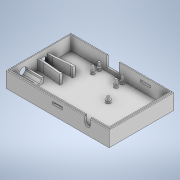
# Autodesk Inventor part: Housing
Saved by Autodesk Inventor 2020 (Build 240168000, 168)
## iProperties
Created: 2019-10-15
Part Number: Housing
Material: Generic
Document SubType Name: Modeling
Designer: strom
Density: 1 g/cm^3
Appearance: Default
Author: strom
Autodesk Inventor part; units mm, degrees
ref_plane "YZ Plane" through (0, 0, 0) normal (1, 0, 0) x (0, 1, 0)
ref_plane "XZ Plane" through (0, 0, 0) normal (0, 1, 0) x (-1, 0, 0)
ref_plane "XY Plane" through (0, 0, 0) normal (0, 0, 1) x (1, 0, 0)
sketch "Sketch1" plane through (0, 0, 0) normal (0, 1, 0) x (-1, 0, 0)
  line L0 (68.58, -43.18) -> (-68.58, -43.18)
  line L1 (-68.58, -43.18) -> (-68.58, 43.18)
  line L2 (-68.58, 43.18) -> (68.58, 43.18)
  line L3 (68.58, 43.18) -> (68.58, -43.18)
  line L4 (96.012, 0) -> (-96.012, 0) projected
  line L5 (0, -60.452) -> (0, 60.452) projected
  point P0 (0, 0)
  dimension "d0" = 137.16
  dimension "d1" = 86.36
  constraints: 8 end point, 2 parallel, 1 horizontal, 1 perpendicular, 2 other
  measures "d0" distance of L1.end L2.end
  measures "d1" distance of L0.end L1.end
extrude "Extrusion1" add sketch "Sketch1" along normal blind 21.59
shell "Shell1" thickness 2.54 removed faces 1 at (-22.86, 21.59, -14.3933)
sketch "Sketch2" plane through (-66.04, 2.54, 40.64) normal (0, 1, 0) x (1, 0, 0)
  line L0 (-29.972, 40.64) -> (162.052, 40.64) projected
  line L1 (66.04, 101.092) -> (66.04, -19.812) projected
  circle A0 centre (83.82, 47.2821) radius 3.175
  circle A1 centre (127, 47.2821) radius 3.175
  circle A2 centre (83.82, 4.1021) radius 3.175
  circle A3 centre (127, 4.1021) radius 3.175
  line L2 (132.08, 0) -> (0, 0) projected
  line L3 (132.08, 81.28) -> (132.08, 0) projected
  point P0 (66.04, 40.64)
  dimension "d5" = 6.35
  dimension "d6" = 6.35
  dimension "d7" = 6.35
  dimension "d8" = 6.35
  dimension "d9" = 43.18
  dimension "d10" = 43.18
  dimension "d11" = 4.1021
  dimension "d22" = 5.08
  constraints: 4 centre point, 2 horizontal alignment, 2 vertical alignment
  measures "d5" diameter of A0
  measures "d6" diameter of A1
  measures "d7" diameter of A3
  measures "d8" diameter of A2
  measures "d9" distance of A1.centre A0.centre
  measures "d10" distance of A2.centre A0.centre
  measures "d11" distance from line of L2 A2.centre
  measures "d22" distance from line of L3 A1.centre
extrude "Extrusion2" add sketch "Sketch2" along normal blind 3.048 contours A0 | A1 | A2 | A3
sketch "Sketch3" plane through (17.78, 5.588, -6.6421) normal (0, 1, 0) x (1, 0, 0)
  circle A0 centre (0, 0) radius 3.175 projected
  circle A1 centre (43.18, 0) radius 3.175 projected
  circle A2 centre (43.18, -43.18) radius 3.175 projected
  circle A3 centre (0, -43.18) radius 3.175 projected
  circle A4 centre (0, 0) radius 3.175 projected
  circle A5 centre (0, 0) radius 1.524
  circle A6 centre (43.18, 0) radius 1.524
  circle A7 centre (0, -43.18) radius 3.175 projected
  circle A8 centre (0, -43.18) radius 1.524
  circle A9 centre (43.18, -43.18) radius 1.524
  point P0 (-17.78, -6.6421)
  dimension "d14" = 3.048
  dimension "d15" = 3.048
  dimension "d16" = 3.048
  dimension "d17" = 3.048
  constraints: 4 centre point, 4 coincident
  measures "d14" diameter of A5
  measures "d15" diameter of A6
  measures "d16" diameter of A9
  measures "d17" diameter of A8
extrude "Extrusion3" add sketch "Sketch3" along normal blind 3.81 contours A5 | A6 | A8 | A9
sketch "Sketch4" plane through (-68.58, 0, 43.18) normal (0, 0, 1) x (1, 0, 0)
  line L0 (89.535, 5.588) -> (83.185, 5.588) projected
  line L1 (83.185, 2.54) -> (89.535, 2.54) projected
  line L2 (132.715, 5.588) -> (126.365, 5.588) projected
  line L3 (126.365, 2.54) -> (132.715, 2.54) projected
  circle A0 centre (108.6485, 13.208) radius 3.6195
  line L4 (87.884, 9.398) -> (84.836, 9.398) projected
  line L5 (84.836, 5.588) -> (87.884, 5.588) projected
  line L6 (128.016, 5.588) -> (131.064, 5.588) projected
  line L7 (131.064, 9.398) -> (128.016, 9.398) projected
  line L8 (128.016, 5.588) -> (131.064, 5.588) projected
  line L9 (105.029, 13.208) -> (105.029, 21.59)
  line L10 (112.268, 13.208) -> (112.268, 21.59)
  line L11 (0, 21.59) -> (137.16, 21.59) projected
  point P0 (68.58, 0)
  dimension "d20" = 7.239
  dimension "d23" = 20.7645
  dimension "d24" = 7.62
  constraints: 4 end point, 2 point on circle, 2 point on line, 2 tangent, 2 vertical, 1 centre point
  measures "d20" diameter of A0
  measures "d23" horizontal distance of A0.centre L4.start
  measures "d24" distance from line of A0.centre L0
extrude "Extrusion4" cut sketch "Sketch4" against normal blind 3.81
sketch "Sketch5" plane through (-66.04, 2.54, 40.64) normal (0, 1, 0) x (1, 0, 0)
  circle A0 centre (127, 4.1021) radius 3.175 projected
  circle A1 centre (127, 47.2821) radius 3.175 projected
  circle A2 centre (83.82, 4.1021) radius 3.175 projected
  circle A3 centre (83.82, 47.2821) radius 3.175 projected
  line L0 (0, 0) -> (132.08, 0) projected
  line L1 (132.08, 0) -> (132.08, 81.28) projected
  line L2 (132.08, 81.28) -> (0, 81.28) projected
  line L3 (0, 81.28) -> (0, 0) projected
  line L4 (0, 25.4) -> (19.05, 25.4)
  line L5 (19.05, 25.4) -> (19.05, 10.16)
  line L6 (19.05, 10.16) -> (0, 10.16)
  line L7 (0, 10.16) -> (0, 25.4)
  line L8 (0, 0) -> (0, 81.28) projected
  point P0 (66.04, 40.64)
  point P1 (0, 25.4)
  point P2 (0, 10.16)
  dimension "d27" = 19.05
  dimension "d28" = 15.24
  dimension "d29" = 10.16
  constraints: 8 end point, 2 parallel, 1 collinear, 1 horizontal, 1 perpendicular
  measures "d27" distance of L5.end L6.end
  measures "d28" distance of L4.end L5.end
  measures "d29" distance between parallel lines of L6 L0
extrude "Extrusion5" add sketch "Sketch5" along normal blind 7.62 contours L3 L4 L5 L6
sketch "Sketch6" plane through (-46.99, 2.54, 30.48) normal (1, 0, 0) x (0, 0, -1)
  line L0 (0, 7.62) -> (15.24, 7.62) projected
  line L1 (5.4106, 2.286) -> (2.286, 5.4106)
  line L2 (2.286, 5.4106) -> (2.286, 9.8294)
  line L3 (2.286, 9.8294) -> (5.4106, 12.954)
  line L4 (5.4106, 12.954) -> (9.8294, 12.954)
  line L5 (9.8294, 12.954) -> (12.954, 9.8294)
  line L6 (12.954, 9.8294) -> (12.954, 5.4106)
  line L7 (12.954, 5.4106) -> (9.8294, 2.286)
  line L8 (9.8294, 2.286) -> (5.4106, 2.286)
  point P0 (30.48, -2.54)
  point P1 (7.62, 7.62)
  dimension "d34" = 10.668
  constraints: 16 end point, 1 horizontal, 1 midpoint, 17 other
  measures "d34" distance between parallel lines of L6 L2
extrude "Extrusion6" cut sketch "Sketch6" against normal through all
sketch "Sketch7" plane through (-46.99, 2.54, 15.24) normal (0, 0, -1) x (-1, 0, 0)
  line L0 (0, 0) -> (19.05, 0) projected
  line L1 (0, 0) -> (0, 7.62) projected
  line L2 (19.05, 7.62) -> (0, 7.62) projected
  line L3 (19.05, 0) -> (19.05, 7.62) projected
  line L4 (0, 0) -> (19.05, 0) projected
  line L5 (2.54, 0) -> (6.35, 0)
  line L6 (6.35, 0) -> (6.35, 1.905)
  line L7 (6.35, 1.905) -> (2.54, 1.905)
  line L8 (2.54, 1.905) -> (2.54, 0)
  line L9 (12.7, 0) -> (16.51, 0)
  line L10 (16.51, 0) -> (16.51, 1.905)
  line L11 (16.51, 1.905) -> (12.7, 1.905)
  line L12 (12.7, 1.905) -> (12.7, 0)
  point P0 (-46.99, -2.54)
  point P1 (16.51, 0)
  point P2 (2.54, 0)
  point P3 (6.35, 0)
  dimension "d37" = 3.81
  dimension "d38" = 1.905
  dimension "d39" = 3.81
  dimension "d40" = 1.905
  dimension "d41" = 2.54
  dimension "d42" = 2.54
  constraints: 16 end point, 4 parallel, 2 horizontal, 2 perpendicular, 2 point on line
  measures "d37" distance of L7.end L6.end
  measures "d38" distance between parallel lines of L0 L7
  measures "d39" distance of L11.end L10.end
  measures "d40" distance of L10.end L9.end
  measures "d41" distance between parallel lines of L10 L3
  measures "d42" distance between parallel lines of L1 L8
extrude "Extrusion7" cut sketch "Sketch7" against normal up to surface (15.24 mm away) contours L8 L7 L6 L0 | L12 L11 L10 L0
sketch "Sketch8" plane through (-66.04, 2.54, 40.64) normal (0, 1, 0) x (1, 0, 0)
  line L0 (0, 81.28) -> (0, 25.4) projected
  line L1 (0, 39.37) -> (7.62, 39.37)
  line L2 (7.62, 39.37) -> (29.718, 37.2111)
  line L3 (29.718, 37.2111) -> (29.718, 37.7191)
  line L4 (29.718, 37.7191) -> (32.258, 37.7191)
  line L5 (32.258, 37.7191) -> (32.258, 34.4108)
  line L6 (32.258, 34.4108) -> (7.4962, 36.83)
  line L7 (7.4962, 36.83) -> (0, 36.83)
  line L8 (0, 49.53) -> (7.62, 49.53)
  line L9 (7.62, 49.53) -> (29.718, 51.6891)
  line L10 (29.718, 51.6891) -> (29.718, 51.1811)
  line L11 (29.718, 51.1811) -> (32.258, 51.1811)
  line L12 (32.258, 51.1811) -> (32.258, 54.4893)
  line L13 (0, 0) -> (0, 81.28) projected
  line L14 (32.258, 54.4893) -> (7.4962, 52.07)
  line L15 (7.4962, 52.07) -> (0, 52.07)
  line L16 (19.05, 25.4) -> (0, 25.4) projected
  point P0 (66.04, 40.64)
  point P1 (0, 54.9166)
  point P2 (0, 54.9166)
  dimension "d45" = 7.62
  dimension "d46" = 7.62
  dimension "d47" = 10.16
  dimension "d48" = 14.478
  dimension "d49" = 22.098
  dimension "d50" = 22.098
  dimension "d51" = 0.508
  dimension "d52" = 0.508
  dimension "d53" = 2.54
  dimension "d54" = 2.54
  dimension "d55" = 2.54
  dimension "d56" = 2.54
  dimension "d57" = 2.54
  dimension "d58" = 2.54
  dimension "d59" = 11.43
  dimension "d60" = 5.58
  constraints: 28 end point, 6 perpendicular, 4 horizontal, 4 point on line, 2 parallel, 1 coincident, 1 vertical, 5 other
  measures "d45" distance of L1.start L1.end
  measures "d46" distance from line of L8.end L0
  measures "d47" distance between parallel lines of L1 L8
  measures "d48" distance of L9.end L2.end
  measures "d49" distance from line of L3 L1.end
  measures "d50" distance from line of L10 L8.end
  measures "d51" distance of L2.end L3.end
  measures "d52" distance of L9.end L10.end
  measures "d53" distance between parallel lines of L1 L7
  measures "d54" distance between parallel lines of L15 L8
  measures "d55" distance between parallel lines of L2 L6
  measures "d56" distance between parallel lines of L14 L9
  measures "d57" distance between parallel lines of L3 L5
  measures "d58" distance between parallel lines of L10 L12
  measures "d59" distance between parallel lines of L16 L7
  measures "d60" angle of L1 L2
extrude "Extrusion8" add sketch "Sketch8" along normal blind 12.7
sketch "Sketch9" plane through (-66.04, 2.54, -40.64) normal (1, 0, 0) x (0, 0, -1)
  line L0 (-41.91, 12.7) -> (-41.91, 0) projected
  line L1 (-31.75, 0) -> (-31.75, 12.7) projected
  circle A0 centre (-36.83, 6.096) radius 5.08
  line L2 (2.54, -2.54) -> (-83.82, -2.54) projected
  point P0 (-40.64, -2.54)
  dimension "d63" = 10.16
  dimension "d64" = 8.636
  constraints: 1 centre point, 1 tangent
  measures "d63" diameter of A0
  measures "d64" distance from line of L2 A0.centre
extrude "Extrusion9" cut sketch "Sketch9" against normal blind 12.7
sketch "Sketch10" plane through (-66.04, 2.54, 40.64) normal (0, 1, 0) x (1, 0, 0)
  line L0 (0, 81.28) -> (132.08, 81.28) projected
  circle A0 centre (40.64, 78.232) radius 2.54
  circle A1 centre (40.64, 69.85) radius 2.54
  circle A2 centre (71.5518, 78.232) radius 2.54
  circle A3 centre (71.5518, 69.85) radius 2.54
  line L1 (0, 0) -> (0, 81.28) projected
  point P0 (66.04, 40.64)
  dimension "d67" = 5.08
  dimension "d68" = 5.08
  dimension "d69" = 5.08
  dimension "d70" = 5.08
  dimension "d71" = 30.9118
  dimension "d72" = 30.9118
  dimension "d73" = 8.382
  dimension "d74" = 8.382
  dimension "d75" = 3.048
  dimension "d76" = 40.64
  constraints: 4 centre point, 1 horizontal alignment, 1 vertical alignment
  measures "d67" diameter of A0
  measures "d68" diameter of A1
  measures "d69" diameter of A2
  measures "d70" diameter of A3
  measures "d71" distance of A2.centre A0.centre
  measures "d72" distance of A3.centre A1.centre
  measures "d73" distance of A0.centre A1.centre
  measures "d74" distance of A3.centre A2.centre
  measures "d75" distance from line of L0 A0.centre
  measures "d76" distance from line of L1 A0.centre
extrude "Extrusion10" add sketch "Sketch10" along normal blind 4.445
sketch "Sketch11" plane through (-66.04, 2.54, -40.64) normal (0, 0, 1) x (1, 0, 0)
  line L0 (43.18, 4.445) -> (38.1, 4.445) projected
  line L1 (38.1, 0) -> (43.18, 0) projected
  line L2 (43.18, 0) -> (43.18, 4.445) projected
  line L3 (38.1, 0) -> (38.1, 4.445) projected
  line L4 (69.0118, 0) -> (69.0118, 4.445) projected
  line L5 (74.0918, 4.445) -> (69.0118, 4.445) projected
  line L6 (74.0918, 0) -> (74.0918, 4.445) projected
  line L7 (47.7139, 5.842) -> (64.4779, 5.842)
  line L8 (64.4779, 5.842) -> (64.4779, 19.05)
  line L9 (64.4779, 19.05) -> (47.7139, 19.05)
  line L10 (47.7139, 19.05) -> (47.7139, 5.842)
  point P0 (66.04, -2.54)
  dimension "d79" = 16.764
  dimension "d80" = 1.397
  dimension "d81" = 13.208
  dimension "d82" = 4.5339
  constraints: 8 end point, 2 parallel, 1 horizontal, 1 perpendicular
  measures "d79" distance of L9.end L8.end
  measures "d80" distance between parallel lines of L7 L5
  measures "d81" distance between parallel lines of L9 L7
  measures "d82" distance between parallel lines of L2 L10
extrude "Extrusion11" cut sketch "Sketch11" against normal blind 3.048 contours L10 L9 L8 L7
sketch "Sketch12" plane through (5.5118, 6.985, -29.21) normal (0, 1, 0) x (1, 0, 0)
  circle A0 centre (-30.9118, 8.382) radius 2.54 projected
  circle A1 centre (-30.9118, 0) radius 2.54 projected
  circle A2 centre (0, 8.382) radius 2.54 projected
  circle A3 centre (0, 0) radius 2.54 projected
  circle A4 centre (-30.9118, 8.382) radius 1.397
  circle A5 centre (-30.9118, 0) radius 2.54 projected
  circle A6 centre (-30.9118, 0) radius 1.397
  circle A7 centre (0, 0) radius 2.54 projected
  circle A8 centre (0, 0) radius 1.397
  circle A9 centre (0, 8.382) radius 1.397
  point P0 (-5.5118, -29.21)
  dimension "d85" = 2.794
  dimension "d86" = 2.794
  dimension "d87" = 2.794
  dimension "d88" = 2.794
  constraints: 4 centre point, 4 coincident
  measures "d85" diameter of A4
  measures "d86" diameter of A6
  measures "d87" diameter of A9
  measures "d88" diameter of A8
extrude "Extrusion12" add sketch "Sketch12" along normal blind 5.08 contours A4 | A6 | A8 | A9
sketch "Sketch13" plane through (0, 21.59, 0) normal (0, 1, 0) x (1, 0, 0)
  line L0 (-18.3261, 40.64) -> (-18.3261, 43.18) projected
  line L1 (-18.3261, 43.18) -> (-68.58, 43.18) projected
  line L2 (-68.58, 43.18) -> (-68.58, -43.18) projected
  line L3 (-68.58, -43.18) -> (36.449, -43.18) projected
  line L4 (36.449, -43.18) -> (36.449, -40.64) projected
  line L5 (36.449, -40.64) -> (-66.04, -40.64) projected
  line L6 (-66.04, -40.64) -> (-66.04, 40.64) projected
  line L7 (-66.04, 40.64) -> (-18.3261, 40.64) projected
  line L8 (-1.5621, 43.18) -> (-1.5621, 40.64) projected
  line L9 (-1.5621, 40.64) -> (66.04, 40.64) projected
  line L10 (66.04, 40.64) -> (66.04, -40.64) projected
  line L11 (66.04, -40.64) -> (43.688, -40.64) projected
  line L12 (43.688, -40.64) -> (43.688, -43.18) projected
  line L13 (43.688, -43.18) -> (68.58, -43.18) projected
  line L14 (68.58, -43.18) -> (68.58, 43.18) projected
  line L15 (68.58, 43.18) -> (-1.5621, 43.18) projected
  line L16 (-67.31, 41.91) -> (67.31, 41.91)
  line L17 (67.31, 41.91) -> (67.31, -41.91)
  line L18 (67.31, -41.91) -> (-67.31, -41.91)
  line L19 (-67.31, -41.91) -> (-67.31, 41.91)
  line L20 (-67.31, 41.91) -> (67.31, -41.91) construction
  line L21 (67.31, 41.91) -> (-67.31, -41.91) construction
  point P0 (0, 0)
  point P1 (-1.5621, 41.91)
  point P2 (43.688, -41.91)
  point P3 (36.449, -41.91)
  point P4 (-18.3261, 41.91)
  dimension "d91" = 1.27
  dimension "d92" = 1.27
  constraints: 12 end point, 2 midpoint, 2 parallel, 1 horizontal, 1 perpendicular
  measures "d91" distance between parallel lines of L18 L13
  measures "d92" distance between parallel lines of L2 L19
extrude "Extrusion13" cut sketch "Sketch13" against normal blind 1.27 contours L16 L19 L18 L4 L3 L2 L1 L0 | L8 L15 L14 L13 L12 L18 L17 L16
draft "FaceDraft1" angle -5 pull direction (0, -1, 0) faces at (1.8627, 21.1667, 41.91) fixed edges at (-15.4305, 20.32, 41.91)
draft "FaceDraft2" angle 5 pull direction (0, 1, 0) fixed plane through (68.1567, 20.32, 13.97) normal (0, 1, 0) faces at (59.436, 20.7433, 41.91)
draft "FaceDraft3" angle 5 pull direction (0, 1, 0) fixed plane through (68.1567, 20.32, 13.97) normal (0, 1, 0) faces at (67.31, 20.7433, 13.933)
draft "FaceDraft4" angle 5 pull direction (0, 1, 0) fixed plane through (68.1567, 20.32, 13.97) normal (0, 1, 0) faces at (44.3156, 20.7433, -41.91)
draft "FaceDraft5" angle 5 pull direction (0, 1, 0) fixed plane through (-33.147, 20.32, 42.7567) normal (0, 1, 0) faces at (-50.982, 21.1667, -41.91)
draft "FaceDraft6" angle 5 pull direction (0, 1, 0) fixed plane through (-33.147, 20.32, 42.7567) normal (0, 1, 0) faces at (-67.31, 20.7433, 13.933)
sketch "Sketch14" plane through (0, 0, 0) normal (1, 0, 0) x (0, 1, 0)
  line L0 (0, -43.18) -> (20.32, -43.18) projected
  line L1 (2.54, -40.64) -> (21.59, -40.64) projected
  line L2 (16.002, -43.18) -> (12.7, -43.18)
  line L3 (12.7, -43.18) -> (12.7, -40.64)
  line L4 (12.7, -40.64) -> (16.002, -40.64)
  line L5 (16.002, -40.64) -> (16.002, -43.18)
  line L6 (21.59, 41.7989) -> (21.59, -41.7989) projected
  line L7 (0, 43.18) -> (20.32, 43.18) projected
  line L8 (2.54, 40.64) -> (21.59, 40.64) projected
  line L9 (16.002, 43.18) -> (12.7, 43.18)
  line L10 (12.7, 43.18) -> (12.7, 40.64)
  line L11 (12.7, 40.64) -> (16.002, 40.64)
  line L12 (16.002, 40.64) -> (16.002, 43.18)
  point P0 (0, 0)
  dimension "d101" = 5.588
  dimension "d102" = 3.302
  dimension "d103" = 5.588
  dimension "d104" = 3.302
  constraints: 16 end point, 4 parallel, 4 point on line, 2 horizontal, 2 perpendicular
  measures "d101" distance between parallel lines of L5 L6
  measures "d102" distance between parallel lines of L5 L3
  measures "d103" distance between parallel lines of L12 L6
  measures "d104" distance between parallel lines of L10 L12
extrude "Extrusion14" cut sketch "Sketch14" against normal mid plane 13.208 contours L7 L12 L8 L10
ref_plane "Work Plane1" through (33.274, 0, 43.18) normal (1, 0, 0) x (0, 0, -1)
sketch "Sketch15" plane through (33.274, 0, 43.18) normal (1, 0, 0) x (0, 0, -1)
  line L0 (83.82, 8.382) -> (83.82, 21.59) projected
  line L1 (86.36, 20.32) -> (86.36, 8.382) projected
  line L2 (83.82, 16.002) -> (86.36, 16.002)
  line L3 (86.36, 16.002) -> (86.36, 12.7)
  line L4 (86.36, 12.7) -> (83.82, 12.7)
  line L5 (83.82, 12.7) -> (83.82, 16.002)
  line L6 (84.9789, 21.59) -> (83.82, 21.59) projected
  point P0 (43.18, 0)
  dimension "d108" = 5.588
  dimension "d109" = 3.302
  constraints: 8 end point, 2 parallel, 2 point on line, 1 horizontal, 1 perpendicular
  measures "d108" distance between parallel lines of L2 L6
  measures "d109" distance between parallel lines of L2 L4
extrude "Extrusion15" cut sketch "Sketch15" against normal mid plane 13.208
sketch "Sketch16" plane through (-18.3261, 8.382, -40.64) normal (0, 1, 0) x (1, 0, 0)
  line L0 (0, 2.54) -> (16.764, 2.54) projected
  line L1 (0, 0) -> (0, 2.54) projected
  line L2 (16.764, 0) -> (0, 0) projected
  line L3 (16.764, 0) -> (16.764, 2.54) projected
  point P0 (18.3261, -40.64)
extrude "Extrusion16" cut sketch "Sketch16" against normal blind 1.27
sketch "Sketch17" plane through (-25.4, 6.985, -29.21) normal (0, 1, 0) x (1, 0, 0)
  circle A0 centre (0, 0) radius 2.54 projected
  circle A1 centre (30.9118, 8.382) radius 2.54 projected
  circle A2 centre (0, 0) radius 2.54 projected
  circle A3 centre (30.9118, 0) radius 2.54 projected
  circle A4 centre (0, 8.382) radius 2.54 projected
  line L0 (-33.02, -20.32) -> (-40.64, -20.32) projected
  line L1 (-40.64, -20.32) -> (-40.64, -30.48) projected
  line L2 (-40.64, -30.48) -> (-33.02, -30.48) projected
  line L3 (-33.02, -30.48) -> (-10.922, -32.6389) projected
  line L4 (-10.922, -32.6389) -> (-10.922, -32.1309) projected
  line L5 (-10.922, -32.1309) -> (-8.382, -32.1309) projected
  line L6 (-8.382, -32.1309) -> (-8.382, -35.4392) projected
  line L7 (-8.382, -35.4392) -> (-33.1438, -33.02) projected
  line L8 (-33.1438, -33.02) -> (-40.64, -33.02) projected
  line L9 (-40.64, -33.02) -> (-40.64, -44.45) projected
  line L10 (-40.64, -44.45) -> (-38.1, -44.45) projected
  line L11 (-38.1, -44.45) -> (-38.1, -59.69) projected
  line L12 (-38.1, -59.69) -> (-40.64, -59.69) projected
  line L13 (-40.64, -59.69) -> (-40.64, -69.85) projected
  line L14 (-40.64, -69.85) -> (91.44, -69.85) projected
  line L15 (91.44, -69.85) -> (91.44, 11.43) projected
  line L16 (91.44, 11.43) -> (-40.64, 11.43) projected
  line L17 (-40.64, 11.43) -> (-40.64, -17.78) projected
  line L18 (-40.64, -17.78) -> (-33.1438, -17.78) projected
  line L19 (-33.1438, -17.78) -> (-8.382, -15.3607) projected
  line L20 (-8.382, -15.3607) -> (-8.382, -18.6689) projected
  line L21 (-8.382, -18.6689) -> (-10.922, -18.6689) projected
  line L22 (-10.922, -18.6689) -> (-10.922, -18.1609) projected
  line L23 (-10.922, -18.1609) -> (-33.02, -20.32) projected
  line L24 (-34.29, -44.45) -> (-27.94, -44.45) projected
  line L25 (-27.94, -44.45) -> (-27.94, -59.69) projected
  line L26 (-27.94, -59.69) -> (-34.29, -59.69) projected
  line L27 (-34.29, -44.45) -> (-34.29, -59.69) projected
  line L28 (-24.13, -44.45) -> (-24.13, -59.69) projected
  line L29 (-24.13, -44.45) -> (-21.59, -44.45) projected
  line L30 (-21.59, -44.45) -> (-21.59, -59.69) projected
  line L31 (-21.59, -59.69) -> (-24.13, -59.69) projected
  circle A5 centre (43.18, -22.5679) radius 3.175 projected
  circle A6 centre (43.18, -65.7479) radius 3.175 projected
  circle A7 centre (86.36, -22.5679) radius 3.175 projected
  circle A8 centre (86.36, -65.7479) radius 3.175 projected
  circle A9 centre (0, 8.382) radius 1.397 projected
  circle A10 centre (0, 0) radius 1.397 projected
  circle A11 centre (30.9118, 0) radius 1.397 projected
  circle A12 centre (30.9118, 8.382) radius 1.397 projected
  point P0 (25.4, -29.21)
extrude "Extrusion17" cut sketch "Sketch17" against normal blind 1.27 contours A0 | A1 | A3 | A4 | A9
equation "\"d6\" = d5"
equation "\"d7\" = d5"
equation "\"d8\" = d5"
equation "\"d15\" = d14"
equation "\"d16\" = d14"
equation "\"d17\" = d14"
equation "\"d46\" = d45"
equation "\"d50\" = d49"
equation "\"d52\" = d51"
equation "\"d54\" = d53"
equation "\"d56\" = d55"
equation "\"d58\" = d57"
equation "\"d68\" = d67"
equation "\"d69\" = d67"
equation "\"d70\" = d67"
equation "\"d72\" = d71"
equation "\"d74\" = d73"
equation "\"d86\" = d85"
equation "\"d87\" = d85"
equation "\"d88\" = d85"
body "Solid1"
